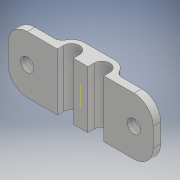
# Autodesk Inventor part: double-ptfe-tube-clip-4mm
Saved by Autodesk Inventor 2018 (Build 220112000, 112)
## iProperties
Created: 2020-01-13
Part Number: double-ptfe-tube-clip-4mm
Material: Generic
Document SubType Name: Modeling
Designer: Vinnie Caprarola
Density: 1 g/cm^3
Appearance: Default
Author: Vinnie Caprarola
Autodesk Inventor part; units mm, degrees
ref_plane "YZ Plane" through (0, 0, 0) normal (1, 0, 0) x (0, 1, 0)
ref_plane "XZ Plane" through (0, 0, 0) normal (0, 1, 0) x (-1, 0, 0)
ref_plane "XY Plane" through (0, 0, 0) normal (0, 0, 1) x (1, 0, 0)
sketch "Sketch1" plane through (0, 0, 0) normal (0, 0, 1) x (1, 0, 0)
  circle A0 centre (0, 0) radius 2.1
  line L0 (-15, 3.4) -> (0, 3.4)
  line L1 (15, 3.4) -> (15, -1.6)
  line L2 (15, -1.6) -> (-15, -1.6)
  line L3 (-15, -1.6) -> (-15, 3.4)
  line L4 (-2.1, 0) -> (-2.1, -1.6)
  line L5 (2.1, 0) -> (2.1, -1.6)
  arc A1 (0, 3.4) -> (-3.0984, 1.4) centre (0, 0) ccw
  line L6 (-15, -1.6) -> (15, -1.6)
  line L7 (15, -1.6) -> (15, 1.4)
  line L8 (15, 1.4) -> (3.0984, 1.4)
  line L9 (-15, 1.4) -> (-15, -1.6)
  line L10 (3.0984, 1.4) -> (-3.0984, 1.4)
  line L11 (-3.0984, 1.4) -> (-15, 1.4)
  line L12 (0, 3.4) -> (15, 3.4)
  arc A2 (3.0984, 1.4) -> (0, 3.4) centre (0, 0) ccw
  arc A3 (-3.0984, 1.4) -> (3.0984, 1.4) centre (0, 0) ccw
  dimension "d0" = 4.2
  dimension "d1" = 30
  dimension "d2" = 5
  dimension "d3" = 1.6
  dimension "d6" = 1.3
  dimension "d7" = 30
  dimension "d8" = 3
  constraints: 26 end point, 8 point on circle, 7 parallel, 5 perpendicular, 4 centre point, 3 horizontal, 2 point on line, 1 coincident, 1 vertical alignment
  measures "d0" diameter of A0
  measures "d1" distance of L0.start L1.start
  measures "d2" distance of L2.end L0.start
  measures "d3" distance from line of point (0, 0) L2
  measures "d6" radial gap between concentric circles of A0 A1
  measures "d7" distance of L9.start L7.end
  measures "d8" distance of L7.end L6.end
extrude "Extrusion1" add sketch "Sketch1" along normal blind 15 contours A0 L10 A3 L2 L5 | A0 L10 A1 A2 | A0 L4 L2 A3 L10 | A2 L12 L1 L8 | L8 L1 L2 A3 | L11 L3 L0 A1 | A3 L2 L3 L11
sketch "Sketch2" plane through (0, 0, 0) normal (0, 0, -1) x (-1, 0, 0)
  line L0 (0, 3.4) -> (-15, 3.4) projected
  arc A0 (0, 3.4) -> (-3.0984, 1.4) centre (0, 0) ccw projected
  line L1 (-15, 1.4) -> (-3.0984, 1.4) projected
  line L2 (-15, 3.4) -> (-15, 1.4)
  line L3 (-15, -1.6) -> (-15, 3.4) projected
  constraints: 2 end point, 1 collinear
extrude "Extrusion2" cut sketch "Sketch2" against normal blind 15
mirror "Mirror1" about plane through (0, 0, 0) normal (1, 0, 0) of "Extrusion2"
thicken "Thicken1" operation add thickness 1 both sides no extend neighbours yes toward (0, -1, 0) faces at (11.0328, 1.4, 5)
thicken "Thicken2" operation add thickness 1 both sides no extend neighbours yes toward (0, -1, 0) faces at (-11.0328, 1.4, 5)
fillet "Fillet1" radius 2 2 edges at (3.3764, 0.4, 7.5) (-3.3764, 0.4, 7.5)
fillet "Fillet2" radius 5 4 edges at (15, -0.6, 15) (15, -0.6, 0) (-15, -0.6, 0) (-15, -0.6, 15)
hole "Hole1" at (10, 0.4, 7.5) direction (0, -1, 0) diameter 3.5 end through all
mirror "Mirror2" about plane through (0, 0, 0) normal (1, 0, 0) of "Hole1"
ref_plane "Work Plane1" through (-4, -1.6, 10) normal (-1, 0, 0) x (0, 0, 1)
split "Split1" plane through (-4, -1.6, 10) removes the side toward (-1, 0, 0)
mirror "Mirror3" about plane through (-4, -1.6, 10) normal (-1, 0, 0)
sketch "Sketch3" plane through (0, 0, 15) normal (0, 0, 1) x (1, 0, 0)
  arc A0 (-4.9543, 1.5111) -> (-11.0457, 1.5111) centre (-8, 0) ccw projected
  line L0 (-8, 3.4) -> (0, 3.4)
  line L1 (0, 3.4) -> (-4, 0)
  line L2 (-4, 0) -> (-8, 3.4)
  point P0 (0, 0)
  constraints: 6 end point, 1 horizontal, 1 point on circle, 1 tangent
extrude "Extrusion3" add sketch "Sketch3" against normal up to surface (15 mm away)
body "Solid1"
